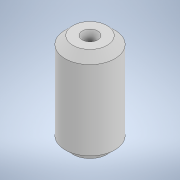
# Autodesk Inventor part: Cate2inchMecanumRoller
Saved by Autodesk Inventor 2020 (Build 240168000, 168)
## iProperties
Created: 2020-01-20
Part Number: Cate2inchMecanumRoller
Material: Generic
Document SubType Name: Modeling
Designer: srini
Density: 1 g/cm^3
Appearance: Default
Author: srini
Autodesk Inventor part; units mm, degrees
ref_plane "YZ Plane" through (0, 0, 0) normal (1, 0, 0) x (0, 1, 0)
ref_plane "XZ Plane" through (0, 0, 0) normal (0, 1, 0) x (-1, 0, 0)
ref_plane "XY Plane" through (0, 0, 0) normal (0, 0, 1) x (1, 0, 0)
sketch "Sketch1" plane through (0, 0, 0) normal (1, 0, 0) x (0, 1, 0)
  line L0 (1.9812, 0) -> (0, 1.9812)
  line L1 (0, 1.9812) -> (0, 4.3743)
  line L2 (0, 4.3743) -> (1.9757, 6.35)
  line L3 (1.9757, 6.35) -> (22.2051, 6.35)
  line L4 (22.2051, 6.35) -> (24.1808, 4.3743)
  line L5 (24.1808, 4.3743) -> (24.1808, 1.9812)
  line L6 (24.1808, 1.9812) -> (22.1996, 0)
  line L7 (22.1996, 0) -> (1.9812, 0)
  point P0 (0, 0)
  dimension "d0" = 6.35
  dimension "d1" = 2.794
  dimension "d2" = 1.9812
  dimension "d3" = 135
  dimension "d4" = 24.1808
  constraints: 17 end point, 7 perpendicular, 2 point on line, 1 parallel, 1 vertical
  measures "d0" distance between parallel lines of L7 L3
  measures "d1" distance of L1.end L2.end
  measures "d2" distance from line of L1 L0.start
  measures "d3" angle of L0 L7
  measures "d4" distance between parallel lines of L1 L5
revolve "Revolution1" add sketch "Sketch1" angle 360 about axis through (0, 22.1996, 0) along (0, -1, 0)
body "Solid1"
